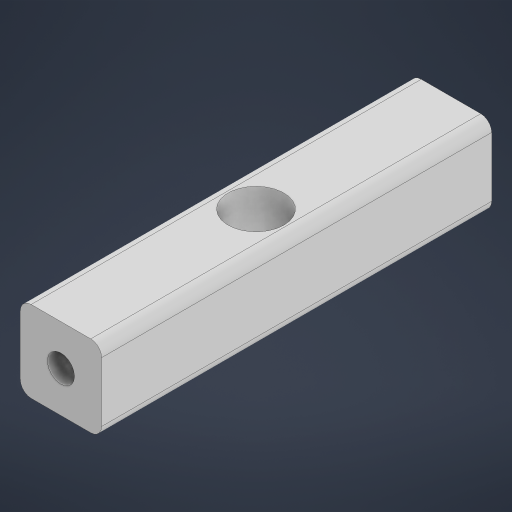
# Autodesk Inventor part: FP V2 Claw Connector
Saved by Autodesk Inventor 2023.6 (Build 276521000, 521)
## iProperties
Created: 2026-02-19
Part Number: FP V2 Claw Connector
Material: Generic
Document SubType Name: Modeling
Designer: user
Density: 1 g/cm^3
Appearance: Default
Author: user
Autodesk Inventor part; units mm, degrees
ref_plane "YZ Plane" through (0, 0, 0) normal (1, 0, 0) x (0, 1, 0)
ref_plane "XZ Plane" through (0, 0, 0) normal (0, 1, 0) x (-1, 0, 0)
sketch "Sketch1" plane through (0, 0, 0) normal (0, 0, 1) x (1, 0, 0)
  line L0 (-7.5, 7.5) -> (7.5, 7.5)
  line L1 (7.5, 7.5) -> (7.5, -7.5)
  line L2 (7.5, -7.5) -> (-7.5, -7.5)
  line L3 (-7.5, -7.5) -> (-7.5, 7.5)
  line L4 (-7.5, 7.5) -> (7.5, -7.5) construction
  line L5 (7.5, 7.5) -> (-7.5, -7.5) construction
  point P0 (0, 0)
  dimension "d0" = 15
  dimension "d1" = 15
  constraints: 12 end point, 2 midpoint, 2 parallel, 1 horizontal, 1 perpendicular
  measures "d0" distance between parallel lines of L1 L3
  measures "d1" distance between parallel lines of L0 L2
extrude "Extrusion1" add sketch "Sketch1" along normal blind 72
sketch "Sketch2" plane through (0, 0, 72) normal (0, 0, 1) x (1, 0, 0)
  circle A0 centre (0, 0) radius 2.5
  dimension "d4" = 5
  constraints: 1 centre point, 1 coincident
  measures "d4" diameter of A0
extrude "Extrusion2" cut sketch "Sketch2" against normal blind 14
ref_plane "Work Plane1" through (0, 0, 36) normal (0, 0, 1) x (1, 0, 0)
mirror "Mirror1" about plane through (0, 0, 36) normal (0, 0, 1) of "Extrusion2"
fillet "Fillet1" radius 2 4 edges at (7.5, 7.5, 36) (-7.5, 7.5, 36) (7.5, -7.5, 36) (-7.5, -7.5, 36)
sketch "Sketch3" plane through (-5.5, 7.5, 0) normal (0, 1, 0) x (1, 0, 0)
  line L0 (-2, -72) -> (-2, 0) projected
  line L1 (-2, -36) -> (13, -36)
  line L2 (13, 0) -> (13, -72) projected
  circle A0 centre (5.5, -36) radius 5.15
  point P0 (5.5, 0)
  dimension "d8" = 10.3
  constraints: 3 midpoint, 2 end point, 1 centre point
  measures "d8" diameter of A0
extrude "Extrusion3" cut sketch "Sketch3" against normal blind 10
body "Solid1"
